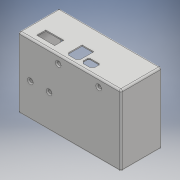
# Autodesk Inventor part: Solar Module Box
Saved by Autodesk Inventor 2017 (Build 210142000, 142)
## iProperties
Created: 2019-06-20
Part Number: Solar Module Box
Material: Generic
Document SubType Name: Modeling
Designer: harneet
Density: 1 g/cm^3
Appearance: Default
Author: harneet
Autodesk Inventor part; units mm, degrees
sketch "Sketch1" plane through (0, 0, 0) normal (0, 1, 0) x (-1, 0, 0)
  line L0 (45, 31) -> (-45, 31)
  line L1 (-45, 31) -> (-45, -31)
  line L2 (-45, -31) -> (45, -31)
  line L3 (45, -31) -> (45, 31)
  point P0 (0, 0)
  dimension "d0" = 90
  dimension "d1" = 62
  dimension "d30" = 45
  dimension "d31" = 31
  constraints: 8 end point, 2 parallel, 1 horizontal, 1 perpendicular
  measures "d0" distance of L2.end L1.end
  measures "d1" distance of L1.end L0.end
  measures "d30" distance from line of point (0, 0) L3
  measures "d31" distance from line of point (0, 0) L0
extrude "Extrusion1" add sketch "Sketch1" along normal blind 36
sketch "Sketch2" plane through (0, 36, 0) normal (0, 1, 0) x (1, 0, 0)
  line L0 (-43.5, 29.5) -> (-43.5, -29.5)
  line L1 (-45, 31) -> (-45, 0) projected
  line L2 (45, 31) -> (-45, 31) projected
  line L3 (45, -31) -> (45, 31) projected
  line L4 (0, -31) -> (45, -31) projected
  line L5 (43.5, 29.5) -> (-43.5, 29.5)
  line L6 (43.5, -29.5) -> (43.5, 29.5)
  line L7 (-43.5, -29.5) -> (43.5, -29.5)
  point P0 (0, 0)
  dimension "d56" = 1.5
  dimension "d57" = 1.5
  dimension "d58" = 1.5
  dimension "d59" = 1.5
  constraints: 8 end point, 2 vertical, 2 other
  measures "d56" distance between parallel lines of L6 L3
  measures "d57" distance between parallel lines of L2 L5
extrude "Extrusion2" cut sketch "Sketch2" against normal blind 34.5
ref_plane "Work Plane1" through (0, 36, 29.5) normal (1, 0, 0) x (0, 0, -1)
ref_plane "Work Plane2" through (-43.5, 36, 0) normal (0, 0, 1) x (1, 0, 0)
sketch "Sketch8" plane through (0, 36, 0) normal (0, 1, 0) x (1, 0, 0)
  line L0 (-43.5, -29.5) -> (-43.5, 29.5) projected
  line L1 (-43.5, 29.5) -> (43.5, 29.5) projected
  line L2 (-43.5, 29.5) -> (-35.5, 29.5)
  line L3 (-35.5, 29.5) -> (-35.5, 21.5)
  line L4 (-35.5, 21.5) -> (-43.5, 21.5)
  line L5 (-43.5, 21.5) -> (-43.5, 29.5)
  line L6 (0, 43.4) -> (0, -43.4) projected
  line L7 (63, 0) -> (-63, 0) projected
  line L8 (43.5, 29.5) -> (35.5, 29.5)
  line L9 (35.5, 29.5) -> (35.5, 21.5)
  line L10 (35.5, 21.5) -> (43.5, 21.5)
  line L11 (43.5, 21.5) -> (43.5, 29.5)
  line L12 (-43.5, -29.5) -> (43.5, -29.5)
  line L13 (-43.5, -29.5) -> (-35.5, -29.5)
  line L14 (-35.5, -29.5) -> (-35.5, -21.5)
  line L15 (-35.5, -21.5) -> (-43.5, -21.5)
  line L16 (-43.5, -21.5) -> (-43.5, -29.5)
  line L17 (43.5, -29.5) -> (35.5, -29.5)
  line L18 (35.5, -29.5) -> (35.5, -21.5)
  line L19 (35.5, -21.5) -> (43.5, -21.5)
  line L20 (43.5, -21.5) -> (43.5, -29.5)
  point P0 (0, 0)
  dimension "d32" = 8
  dimension "d33" = 8
  constraints: 34 end point, 10 symmetric about line, 2 parallel, 1 horizontal, 1 perpendicular
  measures "d32" distance of L3.end L4.end
  measures "d33" distance of L2.end L3.end
extrude "Extrusion5" add sketch "Sketch8" against normal blind 2 contours L1 L11 L10 L9 | L18 L19 L20 L12 | L0 L15 L14 L12 | L0 L1 L3 L4
ref_plane "Work Plane7" through (-43.5, 34, -21.5) normal (0, -0.7071, 0.7071) x (-1, 0, 0)
sketch "Sketch9" plane through (-43.5, 34, -21.5) normal (0, -0.7071, 0.7071) x (-1, 0, 0)
  line L0 (-8, 5.6569) -> (-8, 0) projected
  line L1 (0, 5.6569) -> (0, 0) projected
  line L2 (-8, 5.6569) -> (0, 5.6569) projected
  line L3 (0, 0) -> (-8, 0)
  line L4 (-8, 0) -> (-8, 11)
  line L5 (-8, 11) -> (0, 11)
  line L6 (0, 11) -> (0, 0)
  line L7 (-43.5, -52.3966) -> (-43.5, 44.6184) projected
  line L8 (-87, 0) -> (-79, 0)
  line L9 (-79, 0) -> (-79, 11)
  line L10 (-79, 11) -> (-87, 11)
  line L11 (-87, 11) -> (-87, 0)
  point P0 (-43.5, 8.8388)
  dimension "d37" = 8
  dimension "d38" = 11
  constraints: 16 end point, 4 symmetric about line, 2 parallel, 1 horizontal, 1 perpendicular
  measures "d37" distance between parallel lines of L4 L1
  measures "d38" distance between parallel lines of L3 L5
extrude "Extrusion6" add sketch "Sketch9" against normal up to next
ref_plane "Work Plane8" through (-35.5, 34, 21.5) normal (0, -0.7071, -0.7071) x (1, 0, 0)
sketch "Sketch10" plane through (-35.5, 34, 21.5) normal (0, -0.7071, -0.7071) x (1, 0, 0)
  line L0 (-8, 0) -> (0, 0)
  line L1 (0, 0) -> (0, 11)
  line L2 (0, 11) -> (-8, 11)
  line L3 (-8, 11) -> (-8, 0)
  line L4 (0, -1.4142) -> (-8, -1.4142) projected
  line L5 (0, -1.4142) -> (0, 0) projected
  line L6 (-8, 0) -> (0, 0) projected
  line L7 (-8, -1.4142) -> (-8, 0) projected
  line L8 (0, -31.8198) -> (0, -37.4767) projected
  line L9 (0, -37.4767) -> (71, -37.4767) projected
  line L10 (71, -37.4767) -> (71, -31.8198) projected
  line L11 (71, -31.8198) -> (79, -31.8198) projected
  line L12 (79, -31.8198) -> (79, -1.4142) projected
  line L13 (79, -1.4142) -> (71, -1.4142) projected
  line L14 (71, -1.4142) -> (71, 4.2426) projected
  line L15 (71, 4.2426) -> (0, 4.2426) projected
  line L16 (0, 4.2426) -> (0, -1.4142) projected
  line L17 (0, -1.4142) -> (-8, -1.4142) projected
  line L18 (-8, -1.4142) -> (-8, -31.8198) projected
  line L19 (-8, -31.8198) -> (0, -31.8198) projected
  line L20 (80.5, -38.5373) -> (-9.5, -38.5373) projected
  line L21 (-9.5, -38.5373) -> (-9.5, 5.3033) projected
  line L22 (-9.5, 5.3033) -> (80.5, 5.3033) projected
  line L23 (80.5, 5.3033) -> (80.5, -38.5373) projected
  line L24 (-8, 5.6569) -> (-8, 28.6378) projected
  line L25 (35.5, 53.0684) -> (35.5, -74.6351) projected
  line L26 (79, 0) -> (71, 0)
  line L27 (71, 0) -> (71, 11)
  line L28 (71, 11) -> (79, 11)
  line L29 (79, 11) -> (79, 0)
  line L30 (71, -1.4142) -> (79, -1.4142)
  line L31 (71, -1.4142) -> (71, 0)
  line L32 (79, 0) -> (71, 0)
  line L33 (79, -1.4142) -> (79, 0)
  line L34 (71, 4.2426) -> (71, -1.4142)
  line L35 (71, -1.4142) -> (79, -1.4142)
  point P0 (35.5, 8.8388)
  point P1 (79, 5.6569)
  dimension "d42" = 8
  dimension "d43" = 11
  dimension "d46" = 0
  dimension "d47" = 0
  constraints: 28 end point, 11 symmetric about line, 2 parallel, 1 horizontal, 1 perpendicular
  measures "d42" distance of L0.start L0.end
  measures "d43" distance of L0.end L1.end
  measures "d46" distance between parallel lines of L24 L3
  measures "d47" distance between parallel lines of L0 L6
extrude "Extrusion7" add sketch "Sketch10" against normal up to next contours L3 L22 L1 L0 | L3 L2 L1 L22 | L27 L22 L29 L26 L14 | L27 L28 L29 L22
fillet "Fillet1" radius 2 8 edges at (35.5, 35, 21.5) (35.5, 30.1109, 25.3891) (-35.5, 30.1109, 25.3891) (-35.5, 35, 21.5) (-35.5, 35, -21.5) (35.5, 30.1109, -25.3891) (35.5, 35, -21.5) (-35.5, 30.1109, -25.3891)
sketch "Sketch11" plane through (0, 36, 0) normal (0, 1, 0) x (1, 0, 0)
  circle A0 centre (39, -25) radius 1.75
  line L0 (35.5, -23.5) -> (35.5, -29.5) projected
  line L1 (43.5, -21.5) -> (37.5, -21.5) projected
  line L2 (0, 43.4) -> (0, -43.4) projected
  line L3 (63, 0) -> (-63, 0) projected
  circle A1 centre (-39, -25) radius 1.75
  circle A2 centre (39, 25) radius 1.75
  circle A3 centre (-39, 25) radius 1.75
  point P0 (0, 0)
  dimension "d51" = 3.5
  dimension "d52" = 3.5
  dimension "d53" = 3.5
  constraints: 4 centre point, 3 symmetric about line, 3 other
  measures "d51" diameter of A0
  measures "d52" distance from line of L0 A0.centre
  measures "d53" distance from line of A0.centre L1
extrude "Extrusion8" cut sketch "Sketch11" against normal blind 2.5
fillet "Fillet2" radius 1.5 16 edges at (45, 0, 0) (0, 0, 31) (-45, 0, 0) (0, 0, -31) (45, 18, -31) (45, 36, 0) (45, 18, 31) (0, 36, 31) (0, 36, -31) (-45, 36, 0) (-45, 18, 31) (-45, 18, -31) (40.5, 34, 21.5) (36.0858, 34.2426, 22.0858) (-40.5, 34, 21.5) (-36.0858, 34.2426, 22.0858)
chamfer "Chamfer1" distance 0.5 angle 45 16 edges at (-40.5, 36, -21.5) (-36.0858, 36, -22.0858) (-35.5, 36, -26.5) (-40.5, 36, 21.5) (-36.0858, 36, 22.0858) (-35.5, 36, 26.5) (35.5, 36, 26.5) (36.0858, 36, 22.0858) (40.5, 36, 21.5) (36.0858, 36, -22.0858) (35.5, 36, -26.5) (40.5, 36, -21.5) (37.25, 36, 25) (37.25, 36, -25) (-40.75, 36, -25) (-40.75, 36, 25)
sketch "Sketch12" plane through (-43.5, 34.5, 31) normal (0, 0, 1) x (1, 0, 0)
  line L0 (9.6, -21.3) -> (25.4, -21.3)
  line L1 (25.4, -21.3) -> (25.4, -29.3)
  line L2 (25.4, -29.3) -> (9.6, -29.3)
  line L3 (9.6, -29.3) -> (9.6, -21.3)
  line L4 (0, -34.5) -> (87, -34.5) projected
  line L5 (-1.5, 0) -> (-1.5, -33) projected
  line L6 (36.8, -16.8) -> (36.8, -28.5)
  line L7 (36.8, -28.5) -> (38.8, -30.5)
  line L8 (38.8, -30.5) -> (45.2, -30.5)
  line L9 (45.2, -30.5) -> (47.2, -28.5)
  line L10 (47.2, -28.5) -> (47.2, -16.8)
  line L11 (47.2, -16.8) -> (36.8, -16.8)
  line L12 (51.5003, -30.5) -> (57.5003, -30.5)
  line L13 (57.5003, -30.5) -> (59.5, -28.5003)
  line L14 (57.5003, -30.5) -> (60.3283, -30.5) construction
  line L15 (59.5, -28.5003) -> (59.5, -24.5003)
  line L16 (59.5, -24.5003) -> (58.5006, -23.5)
  line L17 (58.5006, -23.5) -> (50.5006, -23.5)
  line L18 (50.5006, -23.5) -> (49.5, -24.4997)
  line L19 (49.5, -24.4997) -> (49.5, -28.4997)
  line L20 (49.5, -28.4997) -> (51.5003, -30.5)
  point P0 (43.5, -34.5)
  dimension "d64" = 15.8
  dimension "d65" = 8
  dimension "d66" = 5.2
  dimension "d67" = 11.1
  dimension "d68" = 10.4
  dimension "d69" = 11.4
  dimension "d70" = 11.7
  dimension "d71" = 2
  dimension "d73" = 4
  dimension "d74" = 6.4
  dimension "d104" = 6
  dimension "d105" = 2.828
  dimension "d106" = 45
  dimension "d107" = 4
  dimension "d108" = 1.414
  dimension "d109" = 8
  dimension "d110" = 2.3
  dimension "d111" = 10
  dimension "d112" = 4
  dimension "d113" = 7
  dimension "d114" = 4
  constraints: 38 end point, 6 perpendicular, 3 horizontal, 3 parallel, 3 vertical, 1 equal length
  measures "d64" distance of L0.start L0.end
  measures "d65" distance of L2.end L0.start
  measures "d66" distance between parallel lines of L4 L2
  measures "d67" distance between parallel lines of L5 L3
  measures "d68" distance of L10.end L6.start
  measures "d69" distance between parallel lines of L6 L1
  measures "d70" distance of L6.start L6.end
  measures "d71" distance from line of L6.end L8
  measures "d73" distance between parallel lines of L4 L8
  measures "d74" distance of L7.end L8.end
  measures "d104" distance of L12.start L12.end
  measures "d105" distance of L12.end L13.end
  measures "d106" angle of L14 L13
  measures "d107" distance of L13.end L15.end
  measures "d108" distance of L15.end L16.end
  measures "d109" distance of L16.end L17.end
  measures "d110" distance between parallel lines of L19 L10
  measures "d111" distance between parallel lines of L15 L19
  measures "d112" distance between parallel lines of L4 L12
  measures "d113" distance between parallel lines of L12 L17
  measures "d114" distance of L18.end L19.end
extrude "Extrusion9" cut sketch "Sketch12" against normal up to surface (1.5 mm away)
chamfer "Chamfer2" distance 0.5 angle 45 18 edges at (-33.9, 9.2, 29.5) (-26, 5.2, 29.5) (-18.1, 9.2, 29.5) (-26, 13.2, 29.5) (-6.7, 11.85, 29.5) (-5.7, 5, 29.5) (-1.5, 4, 29.5) (3.7, 11.85, 29.5) (2.7, 5, 29.5) (-1.5, 17.7, 29.5) (6, 8.0003, 29.5) (7.0002, 5.0002, 29.5) (11.0003, 4, 29.5) (11.0006, 11, 29.5) (6.5003, 10.5002, 29.5) (15.0002, 4.9998, 29.5) (16, 7.9997, 29.5) (15.5003, 10.4998, 29.5)
sketch "Sketch13" plane through (0, 1.5, 0) normal (0, 1, 0) x (1, 0, 0)
  circle A0 centre (-34.25, 1.498) radius 2.825
  circle A1 centre (-17.75, 1.498) radius 2.825
  circle A2 centre (-32.748, -16) radius 2.825
  circle A3 centre (-19.017, -16) radius 2.825
  circle A4 centre (-9.801, 1.6) radius 2.825
  circle A5 centre (25.551, 1.6) radius 2.825
  circle A6 centre (-9.801, -23.9) radius 2.825
  circle A7 centre (25.551, -23.9) radius 2.825
  line L0 (-43.5, -22) -> (-43.5, 22) projected
  line L1 (36, -29.5) -> (-36, -29.5) projected
  point P0 (0, 0)
  dimension "d120" = 5.65
  dimension "d121" = 5.65
  dimension "d122" = 5.65
  dimension "d123" = 5.65
  dimension "d124" = 5.65
  dimension "d125" = 5.65
  dimension "d126" = 5.65
  dimension "d127" = 5.65
  dimension "d128" = 9.25
  dimension "d129" = 30.998
  dimension "d130" = 16.5
  dimension "d131" = 30.998
  dimension "d132" = 13.731
  dimension "d133" = 10.752
  dimension "d134" = 13.5
  dimension "d135" = 13.5
  dimension "d136" = 25.5
  dimension "d137" = 25.5
  dimension "d138" = 35.352
  dimension "d139" = 33.699
  dimension "d140" = 31.1
  dimension "d141" = 31.1
  dimension "d142" = 5.6
  dimension "d143" = 35.352
  constraints: 8 centre point
  measures "d120" diameter of A0
  measures "d121" diameter of A1
  measures "d122" diameter of A2
  measures "d123" diameter of A3
  measures "d124" diameter of A4
  measures "d125" diameter of A5
  measures "d126" diameter of A6
  measures "d127" diameter of A7
  measures "d128" distance from line of L0 A0.centre
  measures "d129" distance from line of A0.centre L1
  measures "d130" distance of A1.centre A0.centre
  measures "d131" distance from line of L1 A1.centre
  measures "d132" distance of A3.centre A2.centre
  measures "d133" distance from line of A2.centre L0
  measures "d134" distance from line of L1 A2.centre
  measures "d135" distance from line of L1 A3.centre
  measures "d136" distance of A6.centre A4.centre
  measures "d137" distance of A7.centre A5.centre
  measures "d138" distance of A5.centre A4.centre
  measures "d139" distance from line of A4.centre L0
  measures "d140" distance from line of L1 A4.centre
  measures "d141" distance from line of L1 A5.centre
  measures "d142" distance from line of L1 A6.centre
  measures "d143" distance of A7.centre A6.centre
extrude "Extrusion10" add sketch "Sketch13" along normal blind 2.5
sketch "Sketch14" plane through (-17.75, 4, -1.498) normal (0, 1, 0) x (1, 0, 0)
  circle A0 centre (7.949, -25.398) radius 2.825 projected
  circle A1 centre (7.949, 0.102) radius 2.825 projected
  circle A2 centre (-14.998, -17.498) radius 2.825 projected
  circle A3 centre (-16.5, 0) radius 2.825 projected
  circle A4 centre (0, 0) radius 2.825 projected
  circle A5 centre (-1.267, -17.498) radius 2.825 projected
  circle A6 centre (43.301, 0.102) radius 2.825 projected
  circle A7 centre (43.301, -25.398) radius 2.825 projected
  line L0 (61.25, 28.002) -> (61.25, -30.998) projected
  line L1 (-25.75, 28.002) -> (61.25, 28.002) projected
  line L2 (-25.75, -30.998) -> (-25.75, 28.002) projected
  line L3 (61.25, -30.998) -> (-25.75, -30.998) projected
  circle A8 centre (-16.5, 0) radius 1.5
  circle A9 centre (0, 0) radius 1.5
  circle A10 centre (7.949, -25.398) radius 1.5
  circle A11 centre (43.301, -25.398) radius 1.5
  point P0 (17.75, -1.498)
  dimension "d146" = 3
  dimension "d147" = 3
  dimension "d148" = 3
  dimension "d149" = 3
  constraints: 4 centre point, 4 coincident
  measures "d146" diameter of A8
  measures "d147" diameter of A9
  measures "d148" diameter of A10
  measures "d149" diameter of A11
extrude "Extrusion11" cut sketch "Sketch14" against normal up to surface (4 mm away) contours A8 | A9 | A10 | A11
chamfer "Chamfer3" distance 1 angle 45 4 edges at (-11.301, 0, 23.9) (24.051, 0, 23.9) (-19.25, 0, -1.498) (-35.75, 0, -1.498)
fillet "Fillet3" radius 0.25 4 edges at (-35.75, 4, -1.498) (-19.25, 4, -1.498) (-11.301, 4, 23.9) (24.051, 4, 23.9)
chamfer "Chamfer4" distance 1 angle 45 8 edges at (-37.075, 1.5, -1.498) (-20.575, 1.5, -1.498) (-12.626, 1.5, -1.6) (22.726, 1.5, -1.6) (22.726, 1.5, 23.9) (-12.626, 1.5, 23.9) (-21.842, 1.5, 16) (-35.573, 1.5, 16)
equation "\"d30\" = 0.5 * d0"
equation "\"d31\" = 0.5 * d1"
equation "\"d131\" = d129"
body "Solid1"
